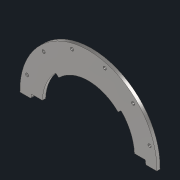
# Autodesk Inventor part: plate1
Saved by Autodesk Inventor 2021 (Build 250183000, 183)
## iProperties
Created: 2021-07-19
Part Number: plate1
Material: 鋼、炭素鋼
Document SubType Name: Sheet Metal
Designer: yuta0
Density: 7.85 g/cm^3
Sheet Metal Rule: Default_mm
Appearance: 半つや出し
Mass: 81.2886 g
Surface Area: 79.4084 cm^2
Volume: 10.3552 cm^3
購入先: Meviy
在庫数: 0.0
Author: yuta0
Autodesk Inventor part; units mm, degrees
ref_plane "YZ Plane" through (0, 0, 0) normal (1, 0, 0) x (0, 1, 0)
ref_plane "XZ Plane" through (0, 0, 0) normal (0, 1, 0) x (-1, 0, 0)
ref_plane "XY Plane" through (0, 0, 0) normal (0, 0, 1) x (1, 0, 0)
sketch "スケッチ5" plane through (0, 0, 3.2) normal (0, 0, 1) x (1, 0, 0)
  circle A0 centre (-16.1762, 60.3704) radius 1.621 projected
  circle A1 centre (16.1762, 60.3704) radius 1.621 projected
  arc A2 (67.5, 0) -> (-67.5, 0) centre (0, 0) ccw projected
  circle A3 centre (-16.1762, 60.3704) radius 5
  circle A4 centre (16.1762, 60.3704) radius 5
  circle A5 centre (-44.1942, 44.1942) radius 1.621 projected
  circle A6 centre (-60.3704, 16.1762) radius 1.621 projected
  circle A7 centre (44.1942, 44.1942) radius 1.621 projected
  circle A8 centre (60.3704, 16.1762) radius 1.621 projected
  arc A9 (62.5, 0) -> (-62.5, 0) centre (0, 0) ccw
  circle A10 centre (-44.1942, 44.1942) radius 5
  circle A11 centre (-60.3704, 16.1762) radius 5
  circle A12 centre (44.1942, 44.1942) radius 5
  circle A13 centre (60.3704, 16.1762) radius 5
  line L0 (-45.5, 0) -> (-67.5, 0) projected
  line L1 (67.5, 0) -> (45.5, 0) projected
  point P0 (17.4703, 65.2)
  point P1 (-17.4703, 65.2)
  point P2 (58.8841, 20.9502)
  point P3 (65.2, 17.4703)
  point P4 (47.7297, 47.7297)
  point P5 (47.5855, 40.52)
  point P6 (40.52, 47.5855)
  point P7 (20.9502, 58.8841)
  point P8 (-65.2, 17.4703)
  point P9 (-58.8841, 20.9502)
  point P10 (-47.5855, 40.52)
  point P11 (-47.7297, 47.7297)
  point P12 (-40.52, 47.5855)
  point P13 (-20.9502, 58.8841)
  point P14 (-11.2987, 61.4702)
  point P15 (11.2987, 61.4702)
  point P16 (61.4702, 11.2987)
  point P17 (-61.4702, 11.2987)
  constraints: 7 centre point, 6 tangent, 3 point on circle
sketch "スケッチ1" plane through (0, 0, 0) normal (0, 0, 1) x (1, 0, 0)
  arc A0 (45.456, 2) -> (-45.5, 0) centre (0, 0) ccw
  arc A1 (67.5, 0) -> (-67.5, 0) centre (0, 0) ccw
  arc A2 (67.4704, -2) -> (-67.4704, -2) centre (0, 0) ccw
  arc A3 (45.456, 2) -> (-45.456, 2) centre (0, 0) ccw
  line L0 (-56.5, 2) -> (-56.5, -2)
  line L1 (-56.5, 2) -> (-45.456, 2)
  line L2 (-56.5, -2) -> (-67.4704, -2)
  line L3 (0, 81.4) -> (0, -15.9)
  line L4 (56.5, 2) -> (56.5, -2)
  line L5 (56.5, 2) -> (45.456, 2)
  line L6 (56.5, -2) -> (67.4704, -2)
  line L7 (-45.5, 0) -> (0, 0)
  point P0 (44.5, 0)
  point P1 (45.5, 0)
  dimension "d0" = 91
  dimension "d1" = 135
  dimension "d58" = 11
  dimension "d61" = 2
  dimension "d62" = 2
  measures "d0" diameter of A0
  measures "d1" diameter of A1
  measures "d58" distance from line of L7.start L0
  measures "d61" distance from line of point (0, 0) L2
  measures "d62" distance from line of L1 L7.end
extrude "プレート2" add sketch "スケッチ1" along normal blind 3.2 contours L1 L0 L2 A2 A1 L3 A0 | L3 A1 A2 L6 L4 L5 A0
sketch "スケッチ2" plane through (0, 0, 3.2) normal (0, 0, 1) x (1, 0, 0)
  circle A0 centre (0, 0) radius 62.5
  point P0 (16.1762, 60.3704)
  point P1 (-16.1762, 60.3704)
  point P2 (-44.1942, 44.1942)
  point P3 (-60.3704, 16.1762)
  point P4 (-60.3704, -16.1762)
  point P5 (-44.1942, -44.1942)
  point P6 (-16.1762, -60.3704)
  point P7 (16.1762, -60.3704)
  point P8 (44.1942, -44.1942)
  point P9 (60.3704, -16.1762)
  point P10 (60.3704, 16.1762)
  point P11 (44.1942, 44.1942)
  dimension "d8" = 125
  dimension "d11" = 360
  dimension "d49" = 0
  constraints: 1 coincident, 16 other
  measures "d49" vertical distance of point (-16.176, 60.37) point (16.176, 60.37)
hole "穴1" at (16.1762, 60.3704, 3.2) at (-16.1762, 60.3704, 3.2) at (-44.1942, 44.1942, 3.2) at (-60.3704, 16.1762, 3.2) at (-60.3704, -16.1762, 3.2) at (-44.1942, -44.1942, 3.2) at (-16.1762, -60.3704, 3.2) at (16.1762, -60.3704, 3.2) at (44.1942, -44.1942, 3.2) at (60.3704, -16.1762, 3.2) at (60.3704, 16.1762, 3.2) at (44.1942, 44.1942, 3.2) direction (0, 0, -1) diameter 3.242 end through all thread size "M4x0.7" class "6H" standard "ANSI Metric M Profile"
sketch "スケッチ6" plane through (0, 0, 3.2) normal (0, 0, 1) x (1, 0, 0)
  line L0 (-32.1734, 32.1734) -> (-29.3449, 29.3449)
  line L1 (29.3449, 29.3449) -> (32.1734, 32.1734)
  line L2 (0, 81.4) -> (0, -15.9) projected
  arc A0 (29.3449, 29.3449) -> (-29.3449, 29.3449) centre (0, 0) ccw
  arc A1 (45.456, 2) -> (-45.456, 2) centre (0, 0) ccw projected
  line L3 (-29.3449, 29.3449) -> (0, 0) construction
  line L4 (0, 0) -> (29.3449, 29.3449) construction
  point P0 (29.3449, 29.3449)
  dimension "d50" = 45
  dimension "d51" = 45
  dimension "d64" = 4
  constraints: 8 end point, 2 point on circle, 1 centre point, 1 collinear, 1 perpendicular
  measures "d50" angle of L2 L0
  measures "d51" angle of L2 L1
  measures "d64" radial gap between concentric circles of A1 A0
extrude "押し出し2" add sketch "スケッチ6" against normal up to surface (3.2 mm away)
fillet "コーナーR7" radius 1 4 edges at (-32.1734, 32.1734, 1.6) (-29.3449, 29.3449, 1.6) (32.1734, 32.1734, 1.6) (29.3449, 29.3449, 1.6)
fillet "コーナーR8" radius 1 4 edges at (-56.5, 2, 1.6) (56.5, 2, 1.6) (-56.5, -2, 1.6) (56.5, -2, 1.6)
equation "\"d18\" = Thickness"
equation "\"d6\" = Thickness"
equation "\"BendRadius\" = Thickness"
equation "\"BendReliefWidth\" = Thickness"
equation "\"BendReliefDepth\" = 0.5 * Thickness"
equation "\"CornerReliefSize\" = 4 * Thickness"
equation "\"MinimumRemnant\" = 2 * Thickness"
equation "\"TransitionRadius\" = BendRadius"
equation "\"JacobiRadiusSize\" = BendRadius"
equation "\"GapSize\" = Thickness"
equation "\"Thickness\" = 3.2"
